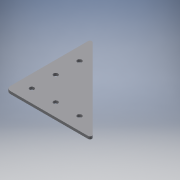
# Autodesk Inventor part: Front Brace
Saved by Autodesk Inventor 2017 (Build 210142000, 142)
## iProperties
Created: 2016-07-21
Part Number: Front Brace
Material: Generic
Document SubType Name: Modeling
Designer: User
Density: 1 g/cm^3
Appearance: Default
Author: User
Autodesk Inventor part; units mm, degrees
ref_plane "YZ Plane" through (0, 0, 0) normal (1, 0, 0) x (0, 1, 0)
ref_plane "XZ Plane" through (0, 0, 0) normal (0, 1, 0) x (-1, 0, 0)
ref_plane "XY Plane" through (0, 0, 0) normal (0, 0, 1) x (1, 0, 0)
sketch "Sketch1" plane through (0, 0, 0) normal (0, 0, 1) x (1, 0, 0)
  line L0 (327.1886, 449.1983) -> (327.071, 449.5859)
  line L1 (327.071, 449.5859) -> (326.8796, 449.944)
  line L2 (326.8796, 449.944) -> (326.6221, 450.2578)
  line L3 (326.6221, 450.2578) -> (233.6862, 543.1798)
  line L4 (233.6862, 543.1798) -> (233.3723, 543.4374)
  line L5 (233.3723, 543.4374) -> (233.0143, 543.6288)
  line L6 (233.0143, 543.6288) -> (232.6258, 543.7467)
  line L7 (232.6258, 543.7467) -> (232.2217, 543.7864)
  line L8 (232.2217, 543.7864) -> (231.8177, 543.7467)
  line L9 (231.8177, 543.7467) -> (231.4291, 543.6288)
  line L10 (231.4291, 543.6288) -> (231.0711, 543.4374)
  line L11 (231.0711, 543.4374) -> (230.7573, 543.1799)
  line L12 (230.7573, 543.1799) -> (230.4997, 542.866)
  line L13 (230.4997, 542.866) -> (230.3083, 542.508)
  line L14 (230.3083, 542.508) -> (230.1905, 542.1195)
  line L15 (230.1905, 542.1195) -> (230.1507, 541.7154)
  line L16 (230.1507, 541.7154) -> (230.1507, 451.7154)
  line L17 (230.1507, 451.7154) -> (230.1934, 451.0627)
  line L18 (230.1934, 451.0627) -> (230.321, 450.4213)
  line L19 (230.321, 450.4213) -> (230.5313, 449.802)
  line L20 (230.5313, 449.802) -> (230.8205, 449.2154)
  line L21 (230.8205, 449.2154) -> (231.1839, 448.6716)
  line L22 (231.1839, 448.6716) -> (231.6151, 448.1799)
  line L23 (231.6151, 448.1799) -> (232.1069, 447.7486)
  line L24 (232.1069, 447.7486) -> (232.6507, 447.3853)
  line L25 (232.6507, 447.3853) -> (233.2372, 447.096)
  line L26 (233.2372, 447.096) -> (233.8566, 446.8858)
  line L27 (233.8566, 446.8858) -> (234.498, 446.7582)
  line L28 (234.498, 446.7582) -> (235.1507, 446.7154)
  line L29 (235.1507, 446.7154) -> (325.1506, 446.7154)
  line L30 (325.1506, 446.7154) -> (325.5547, 446.7551)
  line L31 (325.5547, 446.7551) -> (325.9476, 446.8743)
  line L32 (325.9476, 446.8743) -> (326.3056, 447.0657)
  line L33 (326.3056, 447.0657) -> (326.6195, 447.3233)
  line L34 (326.6195, 447.3233) -> (326.877, 447.6371)
  line L35 (326.877, 447.6371) -> (327.0684, 447.9951)
  line L36 (327.0684, 447.9951) -> (327.1863, 448.3837)
  line L37 (327.1863, 448.3837) -> (327.2275, 448.8028)
  line L38 (327.2275, 448.8028) -> (327.1886, 449.1983)
  line L39 (302.5802, 462.3669) -> (302.3285, 462.9747)
  line L40 (302.3285, 462.9747) -> (301.928, 463.4966)
  line L41 (301.928, 463.4966) -> (301.4061, 463.8971)
  line L42 (301.4061, 463.8971) -> (300.7984, 464.1488)
  line L43 (300.7984, 464.1488) -> (300.1461, 464.2347)
  line L44 (300.1461, 464.2347) -> (299.4939, 464.1489)
  line L45 (299.4939, 464.1489) -> (298.8861, 463.8972)
  line L46 (298.8861, 463.8972) -> (298.3642, 463.4967)
  line L47 (298.3642, 463.4967) -> (297.9637, 462.9748)
  line L48 (297.9637, 462.9748) -> (297.7119, 462.367)
  line L49 (297.7119, 462.367) -> (297.6261, 461.7148)
  line L50 (297.6261, 461.7148) -> (297.7119, 461.0625)
  line L51 (297.7119, 461.0625) -> (297.9636, 460.4548)
  line L52 (297.9636, 460.4548) -> (298.3641, 459.9328)
  line L53 (298.3641, 459.9328) -> (298.886, 459.5323)
  line L54 (298.886, 459.5323) -> (299.4937, 459.2806)
  line L55 (299.4937, 459.2806) -> (300.1459, 459.1948)
  line L56 (300.1459, 459.1948) -> (300.7982, 459.2805)
  line L57 (300.7982, 459.2805) -> (301.406, 459.5323)
  line L58 (301.406, 459.5323) -> (301.9279, 459.9327)
  line L59 (301.9279, 459.9327) -> (302.3284, 460.4546)
  line L60 (302.3284, 460.4546) -> (302.5801, 461.0624)
  line L61 (302.5801, 461.0624) -> (302.666, 461.7147)
  line L62 (302.666, 461.7147) -> (302.5802, 462.3669)
  line L63 (247.5897, 517.3681) -> (247.338, 517.9759)
  line L64 (247.338, 517.9759) -> (246.9375, 518.4978)
  line L65 (246.9375, 518.4978) -> (246.4156, 518.8983)
  line L66 (246.4156, 518.8983) -> (245.8078, 519.15)
  line L67 (245.8078, 519.15) -> (245.1556, 519.2359)
  line L68 (245.1556, 519.2359) -> (244.5033, 519.1501)
  line L69 (244.5033, 519.1501) -> (243.8956, 518.8984)
  line L70 (243.8956, 518.8984) -> (243.3736, 518.4979)
  line L71 (243.3736, 518.4979) -> (242.9731, 517.976)
  line L72 (242.9731, 517.976) -> (242.7214, 517.3683)
  line L73 (242.7214, 517.3683) -> (242.6356, 516.716)
  line L74 (242.6356, 516.716) -> (242.7213, 516.0638)
  line L75 (242.7213, 516.0638) -> (242.9731, 515.456)
  line L76 (242.9731, 515.456) -> (243.3736, 514.9341)
  line L77 (243.3736, 514.9341) -> (243.8954, 514.5336)
  line L78 (243.8954, 514.5336) -> (244.5032, 514.2818)
  line L79 (244.5032, 514.2818) -> (245.1554, 514.196)
  line L80 (245.1554, 514.196) -> (245.8077, 514.2817)
  line L81 (245.8077, 514.2817) -> (246.4154, 514.5335)
  line L82 (246.4154, 514.5335) -> (246.9373, 514.9339)
  line L83 (246.9373, 514.9339) -> (247.3379, 515.4559)
  line L84 (247.3379, 515.4559) -> (247.5896, 516.0636)
  line L85 (247.5896, 516.0636) -> (247.6755, 516.7159)
  line L86 (247.6755, 516.7159) -> (247.5897, 517.3681)
  line L87 (275.0808, 462.367) -> (274.8291, 462.9747)
  line L88 (274.8291, 462.9747) -> (274.4286, 463.4966)
  line L89 (274.4286, 463.4966) -> (273.9067, 463.8971)
  line L90 (273.9067, 463.8971) -> (273.2989, 464.1489)
  line L91 (273.2989, 464.1489) -> (272.6467, 464.2347)
  line L92 (272.6467, 464.2347) -> (271.9945, 464.149)
  line L93 (271.9945, 464.149) -> (271.3867, 463.8972)
  line L94 (271.3867, 463.8972) -> (270.8647, 463.4967)
  line L95 (270.8647, 463.4967) -> (270.4643, 462.9749)
  line L96 (270.4643, 462.9749) -> (270.2125, 462.3671)
  line L97 (270.2125, 462.3671) -> (270.1267, 461.7149)
  line L98 (270.1267, 461.7149) -> (270.2124, 461.0626)
  line L99 (270.2124, 461.0626) -> (270.4642, 460.4549)
  line L100 (270.4642, 460.4549) -> (270.8646, 459.9329)
  line L101 (270.8646, 459.9329) -> (271.3865, 459.5324)
  line L102 (271.3865, 459.5324) -> (271.9943, 459.2807)
  line L103 (271.9943, 459.2807) -> (272.6465, 459.1948)
  line L104 (272.6465, 459.1948) -> (273.2987, 459.2806)
  line L105 (273.2987, 459.2806) -> (273.9065, 459.5323)
  line L106 (273.9065, 459.5323) -> (274.4285, 459.9328)
  line L107 (274.4285, 459.9328) -> (274.829, 460.4547)
  line L108 (274.829, 460.4547) -> (275.0807, 461.0625)
  line L109 (275.0807, 461.0625) -> (275.1665, 461.7146)
  line L110 (275.1665, 461.7146) -> (275.0808, 462.367)
  line L111 (247.5813, 462.367) -> (247.3296, 462.9748)
  line L112 (247.3296, 462.9748) -> (246.9291, 463.4967)
  line L113 (246.9291, 463.4967) -> (246.4072, 463.8972)
  line L114 (246.4072, 463.8972) -> (245.7994, 464.1489)
  line L115 (245.7994, 464.1489) -> (245.1472, 464.2348)
  line L116 (245.1472, 464.2348) -> (244.495, 464.149)
  line L117 (244.495, 464.149) -> (243.8872, 463.8973)
  line L118 (243.8872, 463.8973) -> (243.3653, 463.4968)
  line L119 (243.3653, 463.4968) -> (242.9648, 462.9749)
  line L120 (242.9648, 462.9749) -> (242.713, 462.3671)
  line L121 (242.713, 462.3671) -> (242.6272, 461.7149)
  line L122 (242.6272, 461.7149) -> (242.713, 461.0627)
  line L123 (242.713, 461.0627) -> (242.9647, 460.4549)
  line L124 (242.9647, 460.4549) -> (243.3652, 459.933)
  line L125 (243.3652, 459.933) -> (243.8871, 459.5325)
  line L126 (243.8871, 459.5325) -> (244.4948, 459.2808)
  line L127 (244.4948, 459.2808) -> (245.147, 459.1949)
  line L128 (245.147, 459.1949) -> (245.7993, 459.2807)
  line L129 (245.7993, 459.2807) -> (246.4071, 459.5324)
  line L130 (246.4071, 459.5324) -> (246.929, 459.9329)
  line L131 (246.929, 459.9329) -> (247.3295, 460.4548)
  line L132 (247.3295, 460.4548) -> (247.5812, 461.0625)
  line L133 (247.5812, 461.0625) -> (247.6671, 461.7149)
  line L134 (247.6671, 461.7149) -> (247.5813, 462.367)
  line L135 (247.5854, 489.8677) -> (247.3337, 490.4753)
  line L136 (247.3337, 490.4753) -> (246.9332, 490.9973)
  line L137 (246.9332, 490.9973) -> (246.4114, 491.3978)
  line L138 (246.4114, 491.3978) -> (245.8036, 491.6495)
  line L139 (245.8036, 491.6495) -> (245.1514, 491.7354)
  line L140 (245.1514, 491.7354) -> (244.4991, 491.6496)
  line L141 (244.4991, 491.6496) -> (243.8914, 491.3979)
  line L142 (243.8914, 491.3979) -> (243.3694, 490.9974)
  line L143 (243.3694, 490.9974) -> (242.9689, 490.4755)
  line L144 (242.9689, 490.4755) -> (242.7172, 489.8677)
  line L145 (242.7172, 489.8677) -> (242.6313, 489.2155)
  line L146 (242.6313, 489.2155) -> (242.7171, 488.5632)
  line L147 (242.7171, 488.5632) -> (242.9688, 487.9555)
  line L148 (242.9688, 487.9555) -> (243.3693, 487.4335)
  line L149 (243.3693, 487.4335) -> (243.8912, 487.033)
  line L150 (243.8912, 487.033) -> (244.499, 486.7813)
  line L151 (244.499, 486.7813) -> (245.1512, 486.6954)
  line L152 (245.1512, 486.6954) -> (245.8034, 486.7812)
  line L153 (245.8034, 486.7812) -> (246.4112, 487.0329)
  line L154 (246.4112, 487.0329) -> (246.9331, 487.4334)
  line L155 (246.9331, 487.4334) -> (247.3336, 487.9553)
  line L156 (247.3336, 487.9553) -> (247.5853, 488.563)
  line L157 (247.5853, 488.563) -> (247.6712, 489.2153)
  line L158 (247.6712, 489.2153) -> (247.5854, 489.8677)
  point P0 (0, 0)
  constraints: 318 end point, 2 perpendicular
extrude "Extrusion1" add sketch "Sketch1" along normal blind 3
sketch "Sketch2" plane through (0, 0, 3) normal (0, 0, 1) x (1, 0, 0)
  line L0 (247.5897, 517.3681) -> (247.6755, 516.7159) projected
  line L1 (247.6755, 516.7159) -> (247.5896, 516.0636) projected
  line L2 (247.5896, 516.0636) -> (247.3379, 515.4559) projected
  line L3 (247.3379, 515.4559) -> (246.9373, 514.9339) projected
  line L4 (246.9373, 514.9339) -> (246.4154, 514.5335) projected
  line L5 (246.4154, 514.5335) -> (245.8077, 514.2817) projected
  line L6 (245.8077, 514.2817) -> (245.1554, 514.196) projected
  line L7 (245.1554, 514.196) -> (244.5032, 514.2818) projected
  line L8 (244.5032, 514.2818) -> (243.8954, 514.5336) projected
  line L9 (243.8954, 514.5336) -> (243.3736, 514.9341) projected
  line L10 (243.3736, 514.9341) -> (242.9731, 515.456) projected
  line L11 (242.9731, 515.456) -> (242.7213, 516.0638) projected
  line L12 (242.7213, 516.0638) -> (242.6356, 516.716) projected
  line L13 (242.6356, 516.716) -> (242.7214, 517.3683) projected
  line L14 (242.7214, 517.3683) -> (242.9731, 517.976) projected
  line L15 (242.9731, 517.976) -> (243.3736, 518.4979) projected
  line L16 (243.3736, 518.4979) -> (243.8956, 518.8984) projected
  line L17 (243.8956, 518.8984) -> (244.5033, 519.1501) projected
  line L18 (244.5033, 519.1501) -> (245.1556, 519.2359) projected
  line L19 (245.1556, 519.2359) -> (245.8078, 519.15) projected
  line L20 (245.8078, 519.15) -> (246.4156, 518.8983) projected
  line L21 (246.4156, 518.8983) -> (246.9375, 518.4978) projected
  line L22 (246.9375, 518.4978) -> (247.338, 517.9759) projected
  line L23 (247.338, 517.9759) -> (247.5897, 517.3681) projected
  line L24 (247.5854, 489.8677) -> (247.6712, 489.2153) projected
  line L25 (247.6712, 489.2153) -> (247.5853, 488.563) projected
  line L26 (247.5853, 488.563) -> (247.3336, 487.9553) projected
  line L27 (247.3336, 487.9553) -> (246.9331, 487.4334) projected
  line L28 (246.9331, 487.4334) -> (246.4112, 487.0329) projected
  line L29 (246.4112, 487.0329) -> (245.8034, 486.7812) projected
  line L30 (245.8034, 486.7812) -> (245.1512, 486.6954) projected
  line L31 (245.1512, 486.6954) -> (244.499, 486.7813) projected
  line L32 (244.499, 486.7813) -> (243.8912, 487.033) projected
  line L33 (243.8912, 487.033) -> (243.3693, 487.4335) projected
  line L34 (243.3693, 487.4335) -> (242.9688, 487.9555) projected
  line L35 (242.9688, 487.9555) -> (242.7171, 488.5632) projected
  line L36 (242.7171, 488.5632) -> (242.6313, 489.2155) projected
  line L37 (242.6313, 489.2155) -> (242.7172, 489.8677) projected
  line L38 (242.7172, 489.8677) -> (242.9689, 490.4755) projected
  line L39 (242.9689, 490.4755) -> (243.3694, 490.9974) projected
  line L40 (243.3694, 490.9974) -> (243.8914, 491.3979) projected
  line L41 (243.8914, 491.3979) -> (244.4991, 491.6496) projected
  line L42 (244.4991, 491.6496) -> (245.1514, 491.7354) projected
  line L43 (245.1514, 491.7354) -> (245.8036, 491.6495) projected
  line L44 (245.8036, 491.6495) -> (246.4114, 491.3978) projected
  line L45 (246.4114, 491.3978) -> (246.9332, 490.9973) projected
  line L46 (246.9332, 490.9973) -> (247.3337, 490.4753) projected
  line L47 (247.3337, 490.4753) -> (247.5854, 489.8677) projected
  line L48 (302.5802, 462.3669) -> (302.666, 461.7147) projected
  line L49 (302.666, 461.7147) -> (302.5801, 461.0624) projected
  line L50 (302.5801, 461.0624) -> (302.3284, 460.4546) projected
  line L51 (302.3284, 460.4546) -> (301.9279, 459.9327) projected
  line L52 (301.9279, 459.9327) -> (301.406, 459.5323) projected
  line L53 (301.406, 459.5323) -> (300.7982, 459.2805) projected
  line L54 (300.7982, 459.2805) -> (300.1459, 459.1948) projected
  line L55 (300.1459, 459.1948) -> (299.4937, 459.2806) projected
  line L56 (299.4937, 459.2806) -> (298.886, 459.5323) projected
  line L57 (298.886, 459.5323) -> (298.3641, 459.9328) projected
  line L58 (298.3641, 459.9328) -> (297.9636, 460.4548) projected
  line L59 (297.9636, 460.4548) -> (297.7119, 461.0625) projected
  line L60 (297.7119, 461.0625) -> (297.6261, 461.7148) projected
  line L61 (297.6261, 461.7148) -> (297.7119, 462.367) projected
  line L62 (297.7119, 462.367) -> (297.9637, 462.9748) projected
  line L63 (297.9637, 462.9748) -> (298.3642, 463.4967) projected
  line L64 (298.3642, 463.4967) -> (298.8861, 463.8972) projected
  line L65 (298.8861, 463.8972) -> (299.4939, 464.1489) projected
  line L66 (299.4939, 464.1489) -> (300.1461, 464.2347) projected
  line L67 (300.1461, 464.2347) -> (300.7984, 464.1488) projected
  line L68 (300.7984, 464.1488) -> (301.4061, 463.8971) projected
  line L69 (301.4061, 463.8971) -> (301.928, 463.4966) projected
  line L70 (301.928, 463.4966) -> (302.3285, 462.9747) projected
  line L71 (302.3285, 462.9747) -> (302.5802, 462.3669) projected
  line L72 (247.5813, 462.367) -> (247.6671, 461.7149) projected
  line L73 (247.6671, 461.7149) -> (247.5812, 461.0625) projected
  line L74 (247.5812, 461.0625) -> (247.3295, 460.4548) projected
  line L75 (247.3295, 460.4548) -> (246.929, 459.9329) projected
  line L76 (246.929, 459.9329) -> (246.4071, 459.5324) projected
  line L77 (246.4071, 459.5324) -> (245.7993, 459.2807) projected
  line L78 (245.7993, 459.2807) -> (245.147, 459.1949) projected
  line L79 (245.147, 459.1949) -> (244.4948, 459.2808) projected
  line L80 (244.4948, 459.2808) -> (243.8871, 459.5325) projected
  line L81 (243.8871, 459.5325) -> (243.3652, 459.933) projected
  line L82 (243.3652, 459.933) -> (242.9647, 460.4549) projected
  line L83 (242.9647, 460.4549) -> (242.713, 461.0627) projected
  line L84 (242.713, 461.0627) -> (242.6272, 461.7149) projected
  line L85 (242.6272, 461.7149) -> (242.713, 462.3671) projected
  line L86 (242.713, 462.3671) -> (242.9648, 462.9749) projected
  line L87 (242.9648, 462.9749) -> (243.3653, 463.4968) projected
  line L88 (243.3653, 463.4968) -> (243.8872, 463.8973) projected
  line L89 (243.8872, 463.8973) -> (244.495, 464.149) projected
  line L90 (244.495, 464.149) -> (245.1472, 464.2348) projected
  line L91 (245.1472, 464.2348) -> (245.7994, 464.1489) projected
  line L92 (245.7994, 464.1489) -> (246.4072, 463.8972) projected
  line L93 (246.4072, 463.8972) -> (246.9291, 463.4967) projected
  line L94 (246.9291, 463.4967) -> (247.3296, 462.9748) projected
  line L95 (247.3296, 462.9748) -> (247.5813, 462.367) projected
  line L96 (275.0808, 462.367) -> (275.1665, 461.7146) projected
  line L97 (275.1665, 461.7146) -> (275.0807, 461.0625) projected
  line L98 (275.0807, 461.0625) -> (274.829, 460.4547) projected
  line L99 (274.829, 460.4547) -> (274.4285, 459.9328) projected
  line L100 (274.4285, 459.9328) -> (273.9065, 459.5323) projected
  line L101 (273.9065, 459.5323) -> (273.2987, 459.2806) projected
  line L102 (273.2987, 459.2806) -> (272.6465, 459.1948) projected
  line L103 (272.6465, 459.1948) -> (271.9943, 459.2807) projected
  line L104 (271.9943, 459.2807) -> (271.3865, 459.5324) projected
  line L105 (271.3865, 459.5324) -> (270.8646, 459.9329) projected
  line L106 (270.8646, 459.9329) -> (270.4642, 460.4549) projected
  line L107 (270.4642, 460.4549) -> (270.2124, 461.0626) projected
  line L108 (270.2124, 461.0626) -> (270.1267, 461.7149) projected
  line L109 (270.1267, 461.7149) -> (270.2125, 462.3671) projected
  line L110 (270.2125, 462.3671) -> (270.4643, 462.9749) projected
  line L111 (270.4643, 462.9749) -> (270.8647, 463.4967) projected
  line L112 (270.8647, 463.4967) -> (271.3867, 463.8972) projected
  line L113 (271.3867, 463.8972) -> (271.9945, 464.149) projected
  line L114 (271.9945, 464.149) -> (272.6467, 464.2347) projected
  line L115 (272.6467, 464.2347) -> (273.2989, 464.1489) projected
  line L116 (273.2989, 464.1489) -> (273.9067, 463.8971) projected
  line L117 (273.9067, 463.8971) -> (274.4286, 463.4966) projected
  line L118 (274.4286, 463.4966) -> (274.8291, 462.9747) projected
  line L119 (274.8291, 462.9747) -> (275.0808, 462.367) projected
  line L120 (327.1886, 449.1983) -> (327.071, 449.5859) projected
  line L121 (327.071, 449.5859) -> (326.8796, 449.944) projected
  line L122 (326.8796, 449.944) -> (326.6221, 450.2578) projected
  line L123 (326.6221, 450.2578) -> (233.6862, 543.1798) projected
  line L124 (233.6862, 543.1798) -> (233.3723, 543.4374) projected
  line L125 (233.3723, 543.4374) -> (233.0143, 543.6288) projected
  line L126 (233.0143, 543.6288) -> (232.6258, 543.7467) projected
  line L127 (232.6258, 543.7467) -> (232.2217, 543.7864) projected
  line L128 (232.2217, 543.7864) -> (231.8177, 543.7467) projected
  line L129 (231.8177, 543.7467) -> (231.4291, 543.6288) projected
  line L130 (231.4291, 543.6288) -> (231.0711, 543.4374) projected
  line L131 (231.0711, 543.4374) -> (230.7573, 543.1799) projected
  line L132 (230.7573, 543.1799) -> (230.4997, 542.866) projected
  line L133 (230.4997, 542.866) -> (230.3083, 542.508) projected
  line L134 (230.3083, 542.508) -> (230.1905, 542.1195) projected
  line L135 (230.1905, 542.1195) -> (230.1507, 541.7154) projected
  line L136 (230.1507, 541.7154) -> (230.1507, 451.7154) projected
  line L137 (230.1507, 451.7154) -> (230.1934, 451.0627) projected
  line L138 (230.1934, 451.0627) -> (230.321, 450.4213) projected
  line L139 (230.321, 450.4213) -> (230.5313, 449.802) projected
  line L140 (230.5313, 449.802) -> (230.8205, 449.2154) projected
  line L141 (230.8205, 449.2154) -> (231.1839, 448.6716) projected
  line L142 (231.1839, 448.6716) -> (231.6151, 448.1799) projected
  line L143 (231.6151, 448.1799) -> (232.1069, 447.7486) projected
  line L144 (232.1069, 447.7486) -> (232.6507, 447.3853) projected
  line L145 (232.6507, 447.3853) -> (233.2372, 447.096) projected
  line L146 (233.2372, 447.096) -> (233.8566, 446.8858) projected
  line L147 (233.8566, 446.8858) -> (234.498, 446.7582) projected
  line L148 (234.498, 446.7582) -> (235.1507, 446.7154) projected
  line L149 (235.1507, 446.7154) -> (325.1506, 446.7154) projected
  line L150 (325.1506, 446.7154) -> (325.5547, 446.7551) projected
  line L151 (325.5547, 446.7551) -> (325.9476, 446.8743) projected
  line L152 (325.9476, 446.8743) -> (326.3056, 447.0657) projected
  line L153 (326.3056, 447.0657) -> (326.6195, 447.3233) projected
  line L154 (326.6195, 447.3233) -> (326.877, 447.6371) projected
  line L155 (326.877, 447.6371) -> (327.0684, 447.9951) projected
  line L156 (327.0684, 447.9951) -> (327.1863, 448.3837) projected
  line L157 (327.1863, 448.3837) -> (327.2275, 448.8028) projected
  line L158 (327.2275, 448.8028) -> (327.1886, 449.1983) projected
  circle A0 centre (300.146, 461.7147) radius 2.4985
  circle A1 centre (272.6467, 461.7148) radius 2.4985
  circle A2 centre (245.1471, 461.7148) radius 2.4984
  circle A3 centre (245.1513, 489.2154) radius 2.4985
  circle A4 centre (245.1555, 516.7159) radius 2.4984
  point P0 (0, 0)
  constraints: 15 tangent, 5 centre point
hole "Hole1" at (245.1555, 516.7159, 3) at (245.1513, 489.2154, 3) at (245.1471, 461.7148, 3) at (272.6467, 461.7148, 3) at (300.146, 461.7147, 3) direction (0, 0, -1) diameter 5.2 end through all
body "Solid1"
